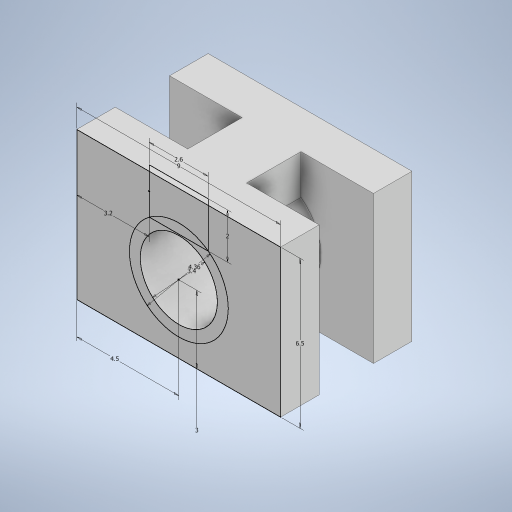
# Autodesk Inventor part: Standard Servo Rubber Grommet
Saved by Autodesk Inventor 2023 (Build 270158000, 158)
## iProperties
Created: 2023-09-05
Part Number: Standard Servo Rubber Grommet
Material: Generic
Document SubType Name: Modeling
Designer: Nate
Density: 1 g/cm^3
Appearance: Default
Author: Nate
Autodesk Inventor part; units mm, degrees
ref_plane "YZ Plane" through (0, 0, 0) normal (1, 0, 0) x (0, 1, 0)
ref_plane "XZ Plane" through (0, 0, 0) normal (0, 1, 0) x (-1, 0, 0)
ref_plane "XY Plane" through (0, 0, 0) normal (0, 0, 1) x (1, 0, 0)
sketch "Sketch1" plane through (0, 0, 0) normal (0, 0, 1) x (1, 0, 0)
  line L0 (0, 0) -> (9, 0)
  line L1 (9, 0) -> (9, 6.5)
  line L2 (9, 6.5) -> (0, 6.5)
  line L3 (0, 6.5) -> (0, 0)
  circle A0 centre (4.5, 3) radius 1.7
  circle A1 centre (4.5, 3) radius 2.18
  line L4 (3.2, 4.75) -> (5.8, 4.75)
  line L5 (5.8, 4.75) -> (5.8, 6.75)
  line L6 (5.8, 6.75) -> (3.2, 6.75)
  line L7 (3.2, 6.75) -> (3.2, 4.75)
  point P0 (3.2, 5.75)
  point P1 (3.2, 6.5)
  point P2 (5.8, 6.5)
  dimension "d5" = 4.36
  dimension "d0" = 9
  dimension "d1" = 6.5
  dimension "d2" = 3.4
  dimension "d3" = 3
  dimension "d4" = 4.5
  dimension "d6" = 2.6
  dimension "d7" = 2
  dimension "d8" = 3.2
  constraints: 16 end point, 4 parallel, 2 horizontal, 2 perpendicular, 1 centre point, 1 coincident, 1 midpoint, 3 other
  measures "d0" distance of L2.end L1.end
  measures "d1" distance of L1.end L0.end
  measures "d2" diameter of A0
  measures "d3" vertical distance of A0.centre L0.start
  measures "d4" horizontal distance of A0.centre L0.start
  measures "d6" distance of L6.end L5.end
  measures "d7" distance of L5.end L4.end
  measures "d8" distance from line of point (3.2, 5.75) L3
extrude "Extrusion1" add sketch "Sketch1" against normal blind 5.8 contours L3 L2 L7 A1 L5 L1 L0 | L2 L5 A1 L7 | L4 A1 | A1 L4 | A0
sketch "Sketch2" plane through (9, 0, 0) normal (1, 0, 0) x (0, 0, -1)
  line L0 (0, 0) -> (5.8, 0) projected
  line L1 (1.7, 0) -> (4.1, 0)
  line L2 (4.1, 0) -> (4.1, 6.5)
  line L3 (4.1, 6.5) -> (1.7, 6.5)
  line L4 (1.7, 6.5) -> (1.7, 0)
  line L5 (0, 0) -> (0, 6.5) projected
  dimension "d11" = 2.4
  dimension "d12" = 6.5
  dimension "d13" = 1.7
  constraints: 8 end point, 2 parallel, 1 horizontal, 1 perpendicular, 1 point on line
  measures "d11" distance of L3.end L2.end
  measures "d12" distance of L2.end L1.end
  measures "d13" distance between parallel lines of L5 L4
extrude "Extrusion2" cut sketch "Sketch2" against normal through all
extrude "Extrusion3" add sketch "Sketch1" against normal blind 5.8 contours L2 L5 A1 L7 | L4 A1 picked at (6.4992, 2.8275)
extrude "Extrusion4" cut sketch "Sketch1" against normal through all contours A0
body "Solid1"
